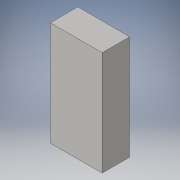
# Autodesk Inventor part: RTS Battery Pack
Saved by Autodesk Inventor 2016 (Build 200138000, 138)
## iProperties
Created: 2016-10-07
Part Number: RTS Battery Pack
Material: Generic
Document SubType Name: Modeling
Designer: sullir
Density: 1 g/cm^3
Appearance: Default
Author: sullir
Autodesk Inventor part; units mm, degrees
ref_plane "YZ Plane" through (0, 0, 0) normal (1, 0, 0) x (0, 1, 0)
ref_plane "XZ Plane" through (0, 0, 0) normal (0, 1, 0) x (-1, 0, 0)
ref_plane "XY Plane" through (0, 0, 0) normal (0, 0, 1) x (1, 0, 0)
sketch "Sketch1" plane through (0, 0, 0) normal (0, 0, 1) x (1, 0, 0)
  line L0 (2.6265, 5.1117) -> (-31.3587, 5.1117)
  line L1 (-31.3587, 5.1117) -> (-31.3587, -63.3159)
  line L2 (-31.3587, -63.3159) -> (2.6265, -63.3159)
  line L3 (2.6265, -63.3159) -> (2.6265, 5.1117)
  point P0 (0, 0)
  dimension "d0" = 68.4276
  dimension "d1" = 33.9852
  constraints: 8 end point, 2 parallel, 1 horizontal, 1 perpendicular
  measures "d0" distance of L2.end L0.start
  measures "d1" distance of L0.start L0.end
extrude "Extrusion1" add sketch "Sketch1" along normal blind 18.034
body "Solid1"
